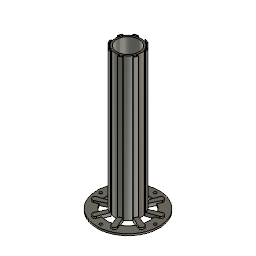
lamp_core by satwik (Autodesk Fusion 360 design; units mm, degrees)
part number: 2026-05-20-20-38-45-437
Autodesk Fusion 360 part; units mm, degrees
sketch "Sketch1" plane through (0, 0, 0) normal (0, 0, 1) x (1, 0, 0)
  circle A0 centre (0, 0) radius 15
  circle A1 centre (0, 0) radius 13
  dimension "d1" = 30
  dimension "d2" = 26
  constraint coincident A0.centre A1.centre
  measures "d1" diameter of A0
  measures "d2" diameter of A1
extrude "Extrude1" add sketch "Sketch1" along normal blind 168
sketch "Sketch2" plane through (0, 0, 168) normal (0, 0, 1) x (-1, 0, 0)
  circle A0 centre (0, 0) radius 13
  circle A1 centre (0, 0) radius 15
  circle A2 centre (0, 0) radius 15
  line L0 (0, 0) -> (0, -29.5553) construction
  line L1 (-4.979, -14.1495) -> (-5.3534, -15.1839)
  line L2 (-6.4858, -13.5253) -> (-6.9525, -14.5214)
  line L3 (-6.9525, -14.5214) -> (-8.3108, -13.8851)
  line L4 (-5.3534, -15.1839) -> (-3.943, -15.6944)
  line L5 (-8.3108, -13.8851) -> (-8.735, -14.7907)
  line L6 (-3.943, -15.6944) -> (-4.2834, -16.6347)
  arc A3 (-8.735, -14.7907) -> (-4.2834, -16.6347) centre (-0.0303, -0.0721) ccw
  line L7 (-6.4858, -13.5253) -> (-4.979, -14.1495)
  line L8 (-5.7324, -13.8374) -> (-8.1748, -19.7332)
  dimension "d5" = 19.9
  dimension "d6" = 25.1
  dimension "d7" = 1.1
  dimension "d8" = 1.1
  dimension "d9" = 1.5
  dimension "d10" = 1.5
  dimension "d11" = 1
  dimension "d12" = 1
  dimension "d16" = 1.631
  dimension "d17" = 3.943
  dimension "d18" = 25.1
  dimension "d19" = 17.1
  constraint coincident A0.centre A1.centre
  constraint vertical L0
  constraint coincident A2 L1.start
  constraint coincident A2 L2.start
  constraint perpendicular L1 L4
  constraint perpendicular L3 L5
  constraint perpendicular L4 L6
  constraint midpoint L7 L8.start
  constraint perpendicular L7 L8
  measures "d5" angle of L0 L1
  measures "d6" angle of L0 L2
  measures "d7" distance of L2.start L2.end
  measures "d8" distance of L1.start L1.end
  measures "d9" distance of L2.end L3.end
  measures "d10" distance of L1.end L4.end
  measures "d11" distance of L3.end L5.end
  measures "d12" distance of L4.end L6.end
  measures "d16" distance of L1.start L2.start
  measures "d17" distance of L0 L4.end
  measures "d18" angle of L0 L5
  measures "d19" radius of A3
extrude "Extrude2" add sketch "Sketch2" along normal blind 168 from surface at -168 contours A1 A2 L2 L3 L5 A3 L8 | A1 A2 L1 L4 L6 A3 L8
sketch "Sketch3" plane through (0, 0, 168) normal (0, 0, 1) x (-1, 0, 0)
  circle A0 centre (0, 0) radius 13
  arc A1 (-4.979, -14.1495) -> (-6.4858, -13.5253) centre (0, 0) ccw
  line L0 (-6.4858, -13.5253) -> (-6.9525, -14.5214)
  line L1 (-6.9525, -14.5214) -> (-8.3108, -13.8851)
  line L2 (-8.3108, -13.8851) -> (-8.735, -14.7907)
  arc A2 (-8.735, -14.7907) -> (-4.2834, -16.6347) centre (-0.0303, -0.0721) ccw
  line L3 (-4.2834, -16.6347) -> (-3.943, -15.6944)
  line L4 (-3.943, -15.6944) -> (-5.3534, -15.1839)
  line L5 (-5.3534, -15.1839) -> (-4.979, -14.1495)
  line L6 (-5.3534, -15.1839) -> (-3.943, -15.6944)
  line L7 (-3.943, -15.6944) -> (-8.6402, -28.6704)
  line L8 (-6.9525, -14.5214) -> (-8.3108, -13.8851)
  line L9 (-8.3108, -13.8851) -> (-14.1648, -26.382)
  arc A3 (-14.1648, -26.382) -> (-8.6402, -28.6704) centre (-11.3916, -27.4999) ccw
  line L10 (-5.3534, -15.1839) -> (-6.9525, -14.5214)
  dimension "d20" = 13.8
  dimension "d22" = 13.8
  dimension "d23" = 2.99
  constraint coincident L4.end L5.start
  constraint coincident L3.end L4.start
  constraint perpendicular L4 L7
  constraint coincident L0.end L1.start
  constraint coincident L1.end L2.start
  constraint perpendicular L1 L9
  measures "d20" distance of L1.end L9.end
  measures "d22" distance of L3.end L7.end
  measures "d23" radius of A3
extrude "Extrude3" add sketch "Sketch3" along normal blind 4 from surface at -168 contours L1 L2 A2 L3 L4 L6 L7 L8 L9 L10 | A2 L7 L9 A3
pattern_circular "C-Pattern1" count 8 over 360 about axis through (0, 0, 1.75) along (0, 0, 1) of "Extrude2", "Extrude3"
sketch "Sketch4" plane through (0, 0, 0) normal (0, 0, 1) x (1, 0, 0)
  circle A0 centre (0, 0) radius 36.6
  circle A1 centre (0, 0) radius 25
  dimension "d29" = 50
  dimension "d30" = 73.2
  constraint coincident A0.centre A1.centre
  constraint concentric A0 A1
  measures "d29" diameter of A1
  measures "d30" diameter of A0
extrude "Extrude4" add sketch "Sketch4" along normal blind 2
sketch "Sketch5" plane through (0, 0, 0) normal (0, 0, 1) x (1, 0, 0)
  circle A0 centre (0, 32) radius 1.6
  dimension "d33" = 3.2
  dimension "d34" = 32
  constraint vertical origin A0.centre
  measures "d33" diameter of A0
  measures "d34" vertical distance of origin A0.centre
extrude "Extrude5" cut sketch "Sketch5" along normal blind 2
pattern_circular "C-Pattern2" count 4 over 360 about axis through (0, 0, 1.75) along (0, 0, 1) of "Extrude5"
